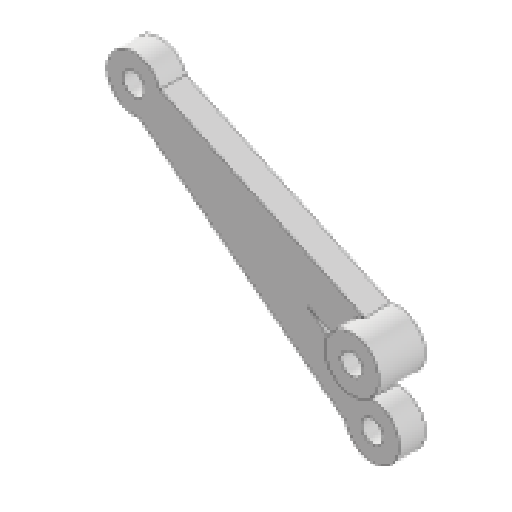
# Autodesk Inventor part: Tip Arm
Saved by Autodesk Inventor 2025 (Build 290162010, 162A)
## iProperties
Created: 2024-11-29
Part Number: Tip Arm
Material: Generic
Document SubType Name: Modeling
Designer: alexa
Density: 1 g/cm^3
Appearance: Default
Author: alexa
Autodesk Inventor part; units mm, degrees
ref_plane "YZ Plane" through (0, 0, 0) normal (1, 0, 0) x (0, 1, 0)
ref_plane "XZ Plane" through (0, 0, 0) normal (0, 1, 0) x (-1, 0, 0)
ref_plane "XY Plane" through (0, 0, 0) normal (0, 0, 1) x (1, 0, 0)
sketch "Sketch1" plane through (0, 0, 0) normal (0, 0, 1) x (1, 0, 0)
  arc A0 (-4.6555, -2.033) -> (-1.4351, 4.8731) centre (0, 0) ccw
  circle A1 centre (0, 0) radius 2.032
  arc A2 (-4.9886, -13.6592) -> (-0.3281, -7.6306) centre (0, -12.7) ccw
  circle A3 centre (0, -12.7) radius 2.032
  line L0 (-43.5629, 16.1615) -> (-4.9886, -13.6592)
  line L1 (-0.3281, -7.6306) -> (-11.9974, 1.3906)
  line L2 (-1.4351, 4.8731) -> (-39.5982, 22.6688)
  arc A4 (-39.5982, 22.6688) -> (-43.5629, 16.1615) centre (-44.45, 21.1635) ccw
  circle A5 centre (-44.45, 21.1635) radius 2.032
  line L3 (-39.5982, 22.6688) -> (-46.4155, 25.8478) construction
  line L4 (-43.5629, 16.1615) -> (-49.5141, 20.7622) construction
  line L5 (-4.6555, -2.033) -> (-11.9974, 1.3906)
  line L6 (0, 0) -> (25.4, 0) construction
  point P0 (-4.1501, -2.9296)
  point P1 (-3.0659, -4.0505)
  dimension "d0" = 10.16
  dimension "d1" = 4.064
  dimension "d7" = 10.16
  dimension "d8" = 4.064
  dimension "d9" = 12.7
  dimension "d10" = 7.62
  dimension "d11" = 3.81
  dimension "d20" = 10.16
  dimension "d21" = 4.064
  dimension "d25" = 7.62
  dimension "d29" = 44.45
  dimension "d30" = 7.62
  dimension "d31" = 3.81
  dimension "d32" = 25.4
  dimension "d33" = 25
  constraints: 14 end point, 8 point on circle, 6 centre point, 4 coincident, 2 collinear, 2 parallel, 1 equal length, 1 horizontal, 1 vertical alignment
  measures "d0" diameter of A0
  measures "d1" diameter of A1
  measures "d7" diameter of A2
  measures "d8" diameter of A3
  measures "d9" distance of point (0, 0) A2.centre
  measures "d10" distance between parallel lines of L0 L1
  measures "d11" distance from line of A2.centre L1
  measures "d20" diameter of A4
  measures "d21" diameter of A5
  measures "d25" distance of L0.start L2.end
  measures "d29" horizontal distance of point (0, 0) A4.centre
  measures "d30" distance between parallel lines of L2 L5
  measures "d31" distance from line of L2 point (0, 0)
  measures "d32" distance of L6.start L6.end
  measures "d33" angle of L6 L2
extrude "Extrusion1" add sketch "Sketch1" along normal blind 4.826
sketch "Sketch4" plane through (0, 0, 4.826) normal (0, 0, 1) x (1, 0, 0)
  arc A0 (-4.6555, -2.033) -> (-1.4351, 4.8731) centre (0, 0) ccw projected
  circle A1 centre (0, 0) radius 2.032 projected
  circle A2 centre (0, 0) radius 5.08
  point P0 (-1.4351, 4.8731)
  point P1 (-3.0659, -4.0505)
  point P2 (5.08, 0)
  point P3 (-1.4351, 4.8731)
  constraints: 1 coincident, 2 other
extrude "Extrusion4" add sketch "Sketch4" along normal blind 3.81
equation "\"d8\" = d1"
equation "\"d11\" = 0.5 * d10"
body "Solid1"
